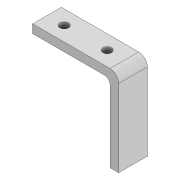
# Autodesk Inventor part: profiletto a l
Saved by Autodesk Inventor 2022 (Build 260153000, 153)
## iProperties
Created: 2025-08-09
Part Number: profiletto a l
Material: Generic
Document SubType Name: Modeling
Designer: sacchie
Density: 1 g/cm^3
Appearance: Default
Author: sacchie
Autodesk Inventor part; units mm, degrees
ref_plane "YZ Plane" through (0, 0, 0) normal (1, 0, 0) x (0, 1, 0)
ref_plane "XZ Plane" through (0, 0, 0) normal (0, 1, 0) x (-1, 0, 0)
ref_plane "XY Plane" through (0, 0, 0) normal (0, 0, 1) x (1, 0, 0)
sketch "Sketch1" plane through (0, 0, 0) normal (0, 0, 1) x (1, 0, 0)
  line L0 (0, -3) -> (0, -30)
  line L1 (0, -30) -> (-3, -30)
  line L2 (-3, 0) -> (-30, 0)
  line L3 (-30, 0) -> (-30, -3)
  line L4 (-30, -3) -> (-5, -3)
  line L5 (-3, -5) -> (-3, -30)
  arc A0 (-3, -5) -> (-5, -3) centre (-5, -5) ccw
  arc A1 (0, -3) -> (-3, 0) centre (-3, -3) ccw
  point P0 (0, 0)
  dimension "d0" = 3
  dimension "d1" = 30
  dimension "d2" = 30
  dimension "d3" = 3
  dimension "d4" = 2
  dimension "d5" = 3
  constraints: 12 end point, 4 perpendicular, 4 point on circle, 4 tangent, 2 centre point, 2 point on line, 1 horizontal, 1 vertical
  measures "d0" distance of L0.end L1.end
  measures "d1" distance of point (0, 0) L0.end
  measures "d2" distance of point (0, 0) L2.end
  measures "d3" distance of L2.end L3.end
  measures "d4" radius of A0
  measures "d5" radius of A1
extrude "Extrusion1" add sketch "Sketch1" along normal blind 10
sketch "Sketch2" plane through (-30, 0, 0) normal (0, 1, 0) x (1, 0, 0)
  line L0 (0, 0) -> (0, -10) projected
  line L1 (0, -5) -> (105.7615, -5) construction
  circle A0 centre (6, -5) radius 1.5
  circle A1 centre (21, -5) radius 1.5
  point P0 (30, 0)
  dimension "d8" = 3
  dimension "d9" = 3
  dimension "d10" = 6
  dimension "d11" = 15
  constraints: 2 centre point, 2 end point, 2 point on line, 1 horizontal, 1 midpoint
  measures "d8" diameter of A1
  measures "d9" diameter of A0
  measures "d10" distance from line of L0 A0.centre
  measures "d11" distance of A0.centre A1.centre
extrude "Extrusion2" cut sketch "Sketch2" against normal blind 3
equation "\"d2\" = d1"
equation "\"d3\" = d0"
equation "\"d9\" = d8"
body "Solid1"
